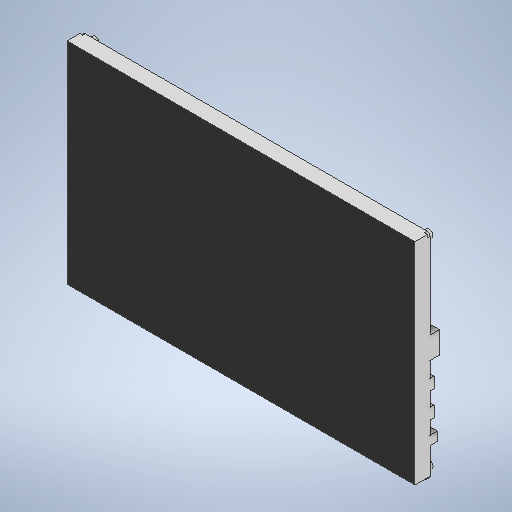
# Autodesk Inventor part: Monitor
Saved by Autodesk Inventor 2025.2 (Build 292293000, 293)
## iProperties
Created: 2025-08-07
Part Number: Monitor
Material: Generic
Document SubType Name: Modeling
Designer: hofma
Density: 1 g/cm^3
Appearance: Default
Author: hofma
Autodesk Inventor part; units mm, degrees
note: some values were not read from the file. Chosen so that the rebuilt part matches the saved one: direction of "Hole2"; direction of "Hole3".
ref_plane "YZ Plane" through (0, 0, 0) normal (1, 0, 0) x (0, 1, 0)
ref_plane "XZ Plane" through (0, 0, 0) normal (0, 1, 0) x (-1, 0, 0)
ref_plane "XY Plane" through (0, 0, 0) normal (0, 0, 1) x (1, 0, 0)
sketch "Sketch1" plane through (0, 0, 0) normal (0, 0, 1) x (1, 0, 0)
  line L0 (-118, 72.5) -> (118, 72.5)
  line L1 (118, 72.5) -> (118, -72.5)
  line L2 (118, -72.5) -> (-118, -72.5)
  line L3 (-118, -72.5) -> (-118, 72.5)
  line L4 (-118, 72.5) -> (118, -72.5) construction
  line L5 (118, 72.5) -> (-118, -72.5) construction
  point P0 (0, 0)
  dimension "d0" = 236
  dimension "d1" = 145
  constraints: 12 end point, 2 midpoint, 2 parallel, 1 horizontal, 1 perpendicular
  measures "d0" distance of L0.start L0.end
  measures "d1" distance of L2.end L0.start
extrude "Extrusion1" add sketch "Sketch1" along normal blind 1.6
fillet "Fillet1" radius 2 4 edges at (-118, 72.5, 0.8) (118, 72.5, 0.8) (118, -72.5, 0.8) (-118, -72.5, 0.8)
sketch "Sketch2" plane through (0, 0, 1.6) normal (0, 0, 1) x (1, 0, 0)
  line L0 (-118, 72.5) -> (118, 72.5)
  line L1 (118, 72.5) -> (118, -70.5)
  line L2 (118, -70.5) -> (-118, -70.5)
  line L3 (-118, -70.5) -> (-118, 72.5)
  line L4 (116, 72.5) -> (-116, 72.5) projected
  line L5 (-118, 70.5) -> (-118, -70.5) projected
  line L6 (118, -70.5) -> (118, 70.5) projected
  point P0 (0, 0)
  point P1 (0, 72.5)
  point P2 (-118, 0)
  point P3 (118, 0)
  dimension "d5" = 143
  constraints: 8 end point, 4 midpoint, 2 parallel, 2 point on line, 1 horizontal, 1 perpendicular
  measures "d5" distance of L2.end L0.start
extrude "Extrusion2" add sketch "Sketch2" along normal blind 8.7
sketch "Sketch3" plane through (0, 0, 0) normal (0, 0, -1) x (-1, 0, 0)
  circle A0 centre (-113.25, 67.75) radius 2.75
  circle A1 centre (113.25, 67.75) radius 2.75
  circle A2 centre (113.25, -67.75) radius 2.75
  circle A3 centre (-113.25, -67.75) radius 2.75
  line L0 (0, 0) -> (49.647, 0) construction
  line L1 (0, 0) -> (0, 39.3254) construction
  line L2 (-116, 72.5) -> (116, 72.5) projected
  line L3 (-118, -70.5) -> (-118, 70.5) projected
  dimension "d8" = 141
  dimension "d9" = 5.5
  dimension "d10" = 4.75
  dimension "d11" = 4.75
  constraints: 4 centre point, 4 end point, 1 horizontal, 1 symmetric about line, 1 vertical, 3 other
  measures "d9" diameter of A0
  measures "d10" distance from line of A0.centre L2
  measures "d11" distance from line of L3 A0.centre
extrude "Extrusion3" add sketch "Sketch3" along normal blind 4
sketch "Sketch5" plane through (113.25, 67.75, -4) normal (0, 0, -1) x (-1, 0, 0)
  circle A0 centre (226.5, 0) radius 2.75 projected
  circle A1 centre (226.5, -135.5) radius 2.75 projected
  circle A2 centre (0, -135.5) radius 2.75 projected
  point P0 (113.25, -67.75)
  point P1 (0, 0)
  constraints: 3 coincident
hole "Hole2" at (113.25, 67.75, -4) at (-113.25, 67.75, -4) at (-113.25, -67.75, -4) at (113.25, -67.75, -4) direction (0, 0, 1) diameter 1.567 depth 4 thread size "M2x0.4" class "6H" standard "ISO Metric profile"
sketch "Sketch6" plane through (0, 0, 0) normal (0, 0, -1) x (-1, 0, 0)
  circle A0 centre (-20, -4.5) radius 2.75
  circle A1 centre (38, -4.5) radius 2.75
  circle A2 centre (-20, -53.5) radius 2.75
  circle A3 centre (38, -53.5) radius 2.75
  line L0 (116, -72.5) -> (-116, -72.5) projected
  line L1 (118, 70.5) -> (118, -70.5) projected
  point P0 (0, 0)
  dimension "d28" = 58
  dimension "d29" = 49
  dimension "d30" = 5.5
  dimension "d31" = 19
  dimension "d32" = 80
  constraints: 4 centre point, 3 equal radius, 2 horizontal alignment, 2 vertical alignment
  measures "d28" distance of A1.centre A0.centre
  measures "d29" distance of A2.centre A0.centre
  measures "d30" diameter of A0
  measures "d31" distance from line of A3.centre L0
  measures "d32" distance from line of L1 A1.centre
extrude "Extrusion4" add sketch "Sketch6" along normal blind 8
sketch "Sketch7" plane through (20, -4.5, -8) normal (0, 0, -1) x (-1, 0, 0)
  circle A0 centre (0, 0) radius 2.75 projected
  circle A1 centre (58, 0) radius 2.75 projected
  circle A2 centre (0, -49) radius 2.75 projected
  circle A3 centre (58, -49) radius 2.75 projected
  point P0 (20, 4.5)
  constraints: 4 coincident
hole "Hole3" at (20, -4.5, -8) at (-38, -4.5, -8) at (20, -53.5, -8) at (-38, -53.5, -8) direction (0, 0, 1) diameter 1.567 depth 8 thread size "M2x0.4" class "6H" standard "ISO Metric profile"
sketch "Sketch8" plane through (0, 0, 0) normal (0, 0, -1) x (-1, 0, 0)
  point P0 (0, 0)
sketch "Sketch9" plane through (0, 0, 0) normal (0, 0, -1) x (-1, 0, 0)
  line L0 (-100, 31.5) -> (-60, 31.5)
  line L1 (-60, 31.5) -> (-60, 59.5)
  line L2 (-60, 59.5) -> (-100, 59.5)
  line L3 (-100, 59.5) -> (-100, 31.5)
  line L4 (-100, 31.5) -> (-60, 59.5) construction
  line L5 (-60, 31.5) -> (-100, 59.5) construction
  line L6 (-116, 72.5) -> (116, 72.5) projected
  line L7 (-118, -70.5) -> (-118, 70.5) projected
  point P0 (0, 0)
  point P1 (-80, 45.5)
  dimension "d42" = 13
  dimension "d43" = 18
  dimension "d44" = 28
  dimension "d45" = 40
  constraints: 12 end point, 2 midpoint, 2 parallel, 1 horizontal, 1 perpendicular
  measures "d42" distance between parallel lines of L6 L2
  measures "d43" distance between parallel lines of L7 L3
  measures "d44" distance of L0.end L1.end
  measures "d45" distance of L0.start L0.end
extrude "Extrusion5" add sketch "Sketch9" along normal blind 10
fillet "Fillet2" radius 5 4 edges at (60, 59.5, -5) (100, 59.5, -5) (100, 31.5, -5) (60, 31.5, -5)
mirror "Mirror1" about plane through (0, 0, 0) normal (1, 0, 0) of "Fillet2", "Extrusion5"
sketch "Sketch10" plane through (0, 0, 0) normal (0, 0, -1) x (-1, 0, 0)
  line L0 (118, 70.5) -> (118, -70.5) projected
  line L1 (118, -7.5) -> (103, -7.5)
  line L2 (103, -7.5) -> (103, -27.5)
  line L3 (103, -27.5) -> (118, -27.5)
  line L4 (118, -27.5) -> (118, -7.5)
  line L5 (116, -72.5) -> (-116, -72.5) projected
  point P0 (0, 0)
  dimension "d49" = 20
  dimension "d50" = 15
  dimension "d51" = 45
  constraints: 8 end point, 2 parallel, 1 horizontal, 1 perpendicular, 1 point on line
  measures "d49" distance between parallel lines of L3 L1
  measures "d50" distance of L1.start L1.end
  measures "d51" distance between parallel lines of L3 L5
extrude "Extrusion6" add sketch "Sketch10" along normal blind 4
sketch "Sketch11" plane through (0, 0, 0) normal (0, 0, -1) x (-1, 0, 0)
  line L0 (-118, -70.5) -> (-118, 72.5) projected
  line L1 (-118, 12.5) -> (-103, 12.5)
  line L2 (-103, 12.5) -> (-103, -2.5)
  line L3 (-103, -2.5) -> (-118, -2.5)
  line L4 (-118, -2.5) -> (-118, 12.5)
  line L5 (116, -72.5) -> (-116, -72.5) projected
  point P0 (0, 0)
  dimension "d54" = 15
  dimension "d55" = 15
  dimension "d56" = 70
  constraints: 8 end point, 2 parallel, 1 horizontal, 1 perpendicular, 1 point on line
  measures "d54" distance of L1.start L1.end
  measures "d55" distance of L1.end L2.end
  measures "d56" distance between parallel lines of L5 L3
extrude "Extrusion7" add sketch "Sketch11" along normal blind 6.3
sketch "Sketch12" plane through (0, 0, 0) normal (0, 0, -1) x (-1, 0, 0)
  line L0 (-118, -70.5) -> (-118, 72.5) projected
  line L1 (-118, -13) -> (-111.5, -13)
  line L2 (-111.5, -13) -> (-111.5, -20.5)
  line L3 (-111.5, -20.5) -> (-118, -20.5)
  line L4 (-118, -20.5) -> (-118, -13)
  line L5 (-118, -30) -> (-111.5, -30)
  line L6 (-111.5, -30) -> (-111.5, -37.5)
  line L7 (-111.5, -37.5) -> (-118, -37.5)
  line L8 (-118, -37.5) -> (-118, -30)
  line L9 (116, -72.5) -> (-116, -72.5) projected
  point P0 (0, 0)
  dimension "d59" = 35
  dimension "d60" = 52
  dimension "d61" = 6.5
  dimension "d62" = 7.5
  constraints: 16 end point, 4 parallel, 3 point on line, 2 horizontal, 2 perpendicular, 1 collinear
  measures "d59" distance between parallel lines of L7 L9
  measures "d60" distance between parallel lines of L3 L9
  measures "d61" distance of L1.start L1.end
  measures "d62" distance of L1.end L2.end
extrude "Extrusion8" add sketch "Sketch12" along normal blind 2.75
sketch "Sketch13" plane through (0, 0, 0) normal (0, 0, -1) x (-1, 0, 0)
  line L0 (-118, -70.5) -> (-118, 72.5) projected
  line L1 (-118, -46.5) -> (-104, -46.5)
  line L2 (-104, -46.5) -> (-104, -52.5)
  line L3 (-104, -52.5) -> (-118, -52.5)
  line L4 (-118, -52.5) -> (-118, -46.5)
  line L5 (116, -72.5) -> (-116, -72.5) projected
  point P0 (0, 0)
  dimension "d65" = 14
  dimension "d66" = 6
  dimension "d67" = 20
  constraints: 8 end point, 2 parallel, 1 horizontal, 1 perpendicular, 1 point on line
  measures "d65" distance of L1.start L1.end
  measures "d66" distance of L1.end L2.end
  measures "d67" distance between parallel lines of L3 L5
extrude "Extrusion9" add sketch "Sketch13" along normal blind 5
equation "\"d11\" = d10"
body "Solid1"
